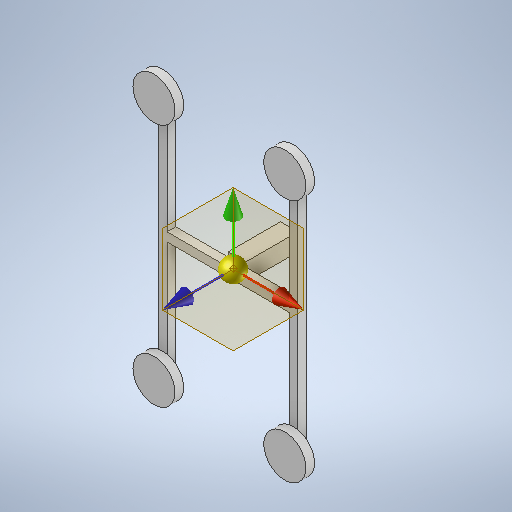
# Autodesk Inventor part: LINK 6
Saved by Autodesk Inventor 2025.4 (Build 294407000, 407)
## iProperties
Created: 2026-03-19
Part Number: LINK 6
Material: Generic
Document SubType Name: Modeling
Designer: dawid
Density: 1 g/cm^3
Appearance: Default
Mass: 2600.51 g
Surface Area: 3253.29 cm^2
Volume: 2600.51 cm^3
Author: dawid
Autodesk Inventor part; units mm, degrees
ref_plane "YZ Plane" through (0, 0, 0) normal (1, 0, 0) x (0, 1, 0)
ref_plane "XZ Plane" through (0, 0, 0) normal (0, 1, 0) x (-1, 0, 0)
ref_plane "XY Plane" through (0, 0, 0) normal (0, 0, 1) x (1, 0, 0)
sketch "Sketch1" plane through (0, 0, 0) normal (0, 0, 1) x (1, 0, 0)
  line L0 (-25, -25) -> (25, -25)
  line L1 (25, -25) -> (25, 25)
  line L2 (25, 25) -> (-25, 25)
  line L3 (-25, 25) -> (-25, -25)
  point P0 (0, 0)
  dimension "d0" = 50
  dimension "d1" = 50
  dimension "d2" = 25
  dimension "d3" = 25
  constraints: 8 end point, 2 parallel, 1 horizontal, 1 perpendicular
  measures "d0" distance of L2.end L1.end
  measures "d1" distance of L1.end L0.end
  measures "d2" distance from line of point (0, 0) L3
  measures "d3" distance from line of point (0, 0) L2
extrude "Extrusion1" add sketch "Sketch1" along normal blind 150
sketch "Sketch2" plane through (0, 0, 0) normal (0, 0, -1) x (-1, 0, 0)
  circle A0 centre (0, 0) radius 5
  dimension "d6" = 10
  constraints: 1 centre point, 1 coincident
  measures "d6" diameter of A0
extrude "Extrusion2" add sketch "Sketch2" along normal blind 10
sketch "Sketch3" plane through (0, 0, 150) normal (0, 0, 1) x (1, 0, 0)
  line L0 (-200, -12.5) -> (0, -12.5)
  line L1 (0, -12.5) -> (0, 12.5)
  line L2 (0, 12.5) -> (-200, 12.5)
  line L3 (-200, 12.5) -> (-200, -12.5)
  line L4 (-200, -350) -> (-175, -350)
  line L5 (-175, -350) -> (-175, 350)
  line L6 (-175, 350) -> (-200, 350)
  line L7 (-200, 350) -> (-200, -350)
  line L8 (200, -12.5) -> (0, -12.5)
  line L9 (0, 12.5) -> (200, 12.5)
  line L10 (200, 12.5) -> (200, -12.5)
  line L11 (200, -350) -> (175, -350)
  line L12 (175, -350) -> (175, 350)
  line L13 (175, 350) -> (200, 350)
  line L14 (200, 350) -> (200, -350)
  point P0 (0, 0)
  point P1 (0, 0)
  point P2 (-187.5, -350)
  point P3 (187.5, -350)
  point P4 (-175, -12.5)
  point P5 (175, -12.5)
  point P6 (175, 12.5)
  point P7 (-175, 12.5)
  dimension "d9" = 25
  dimension "d10" = 200
  dimension "d11" = 25
  dimension "d12" = 700
  dimension "d13" = 350
  constraints: 30 end point, 7 symmetric about line, 4 parallel, 2 horizontal, 2 midpoint, 2 perpendicular, 1 coincident, 1 collinear
  measures "d9" distance of L0.end L1.end
  measures "d10" distance between parallel lines of L1 L3
  measures "d11" distance of L6.end L5.end
  measures "d12" distance of L5.end L4.end
  measures "d13" vertical distance of point (0, 0) point (-187.5, -350)
extrude "Extrusion3" add sketch "Sketch3" along normal blind 25
sketch "Sketch4" plane through (0, 0, 175) normal (0, 0, 1) x (1, 0, 0)
  line L0 (-200, -350) -> (-175, -350) projected
  circle A0 centre (-187.5, -350) radius 60
  line L1 (-187.5, -350) -> (-187.5, 371.532) construction
  line L2 (-187.5, -350) -> (187.5, -350) construction
  line L3 (175, -350) -> (200, -350) projected
  circle A1 centre (-187.5, 350) radius 60
  circle A2 centre (187.5, -350) radius 60
  circle A3 centre (187.5, 350) radius 60
  point P0 (0, 0)
  dimension "d16" = 120
  dimension "d19" = 700
  dimension "d22" = 375
  constraints: 4 centre point, 4 end point, 2 midpoint, 2 vertical, 1 horizontal, 6 other
  measures "d16" diameter of A0
  measures "d19" distance of L1.start A1.centre
  measures "d22" distance of L1.start A2.centre
extrude "Extrusion4" add sketch "Sketch4" along normal blind 25
equation "\"d0\" = d1"
equation "\"d2\" = 0.5 * d0"
equation "\"d3\" = d2"
equation "\"d13\" = 0.5 * d12"
body "Solid1"
